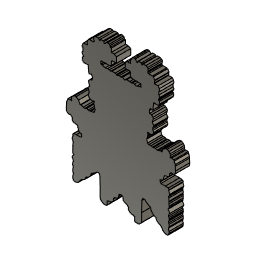
Keychain (Autodesk Fusion 360 design; units mm, degrees)
Autodesk Fusion 360 part; units mm, degrees
sketch "Sketch1" plane through (0, 0, 0) normal (0, 1, 0) x (1, 0, 0)
  line L0 (0.3, -15.5) -> (0.3, -15.9)
  line L1 (0.3, -15.9) -> (0.379, -15.9401)
  line L2 (0.379, -15.9401) -> (0.466, -15.9842)
  line L3 (0.466, -15.9842) -> (0.55, -15.9842)
  line L4 (0.55, -15.9842) -> (0.6648, -15.9842)
  line L5 (0.6648, -15.9842) -> (0.6648, -16.25)
  line L6 (0.6648, -16.25) -> (0.75, -16.25)
  line L7 (0.75, -16.25) -> (0.75, -16.3598)
  line L8 (0.75, -16.3598) -> (0.8165, -16.4115)
  line L9 (0.8165, -16.4115) -> (0.9263, -16.4405)
  line L10 (0.9263, -16.4405) -> (1.007, -16.426)
  line L11 (1.007, -16.426) -> (1.0561, -16.3628)
  line L12 (1.0561, -16.3628) -> (1.1168, -16.2847)
  line L13 (1.1168, -16.2847) -> (1.1655, -16.2759)
  line L14 (1.1655, -16.2759) -> (1.184, -16.3787)
  line L15 (1.184, -16.3787) -> (1.2314, -16.4034)
  line L16 (1.2314, -16.4034) -> (1.35, -16.4034)
  line L17 (1.35, -16.4034) -> (1.43, -16.4034)
  line L18 (1.43, -16.4034) -> (1.4623, -16.3414)
  line L19 (1.4623, -16.3414) -> (1.4623, -16.2775)
  line L20 (1.4623, -16.2775) -> (1.5139, -16.3414)
  line L21 (1.5139, -16.3414) -> (1.5602, -16.3987)
  line L22 (1.5602, -16.3987) -> (1.6237, -16.3987)
  line L23 (1.6237, -16.3987) -> (1.75, -16.3987)
  line L24 (1.75, -16.3987) -> (1.8659, -16.3356)
  line L25 (1.8659, -16.3356) -> (1.9094, -16.2678)
  line L26 (1.9094, -16.2678) -> (1.9094, -16.2)
  line L27 (1.9094, -16.2) -> (1.9094, -16.15)
  line L28 (1.9094, -16.15) -> (1.8726, -16.0823)
  line L29 (1.8726, -16.0823) -> (1.8726, -16.0289)
  line L30 (1.8726, -16.0289) -> (1.9342, -15.9953)
  line L31 (1.9342, -15.9953) -> (2.05, -15.9953)
  line L32 (2.05, -15.9953) -> (2.1322, -15.9953)
  line L33 (2.1322, -15.9953) -> (2.2162, -15.9953)
  line L34 (2.2162, -15.9953) -> (2.2759, -15.974)
  line L35 (2.2759, -15.974) -> (2.305, -15.9304)
  line L36 (2.305, -15.9304) -> (2.3387, -15.8797)
  line L37 (2.3387, -15.8797) -> (2.376, -15.8239)
  line L38 (2.376, -15.8239) -> (2.3574, -15.7715)
  line L39 (2.3574, -15.7715) -> (2.3574, -15.7205)
  line L40 (2.3574, -15.7205) -> (2.3574, -15.65)
  line L41 (2.3574, -15.65) -> (2.3381, -15.5959)
  line L42 (2.3381, -15.5959) -> (2.45, -15.5959)
  line L43 (2.45, -15.5959) -> (2.5213, -15.5959)
  line L44 (2.5213, -15.5959) -> (2.6101, -15.5959)
  line L45 (2.6101, -15.5959) -> (2.694, -15.4671)
  line L46 (2.694, -15.4671) -> (2.7215, -15.304)
  line L47 (2.7215, -15.304) -> (2.6654, -15.2946)
  line L48 (2.6654, -15.2946) -> (2.6654, -15.0651)
  line L49 (2.6654, -15.0651) -> (2.7369, -14.9554)
  line L50 (2.7369, -14.9554) -> (2.6654, -14.8407)
  line L51 (2.6654, -14.8407) -> (2.6201, -14.768)
  line L52 (2.6201, -14.768) -> (2.6428, -14.7332)
  line L53 (2.6428, -14.7332) -> (2.7012, -14.6968)
  line L54 (2.7012, -14.6968) -> (2.7012, -14.5195)
  line L55 (2.7012, -14.5195) -> (2.6315, -14.4076)
  line L56 (2.6315, -14.4076) -> (2.2904, -14.4076)
  line L57 (2.2904, -14.4076) -> (2.25, -13.95)
  line L58 (2.25, -13.95) -> (2.2, -13.9)
  line L59 (2.2, -13.9) -> (2.0693, -13.95)
  line L60 (2.0693, -13.95) -> (2.0337, -13.9)
  line L61 (2.0337, -13.9) -> (1.9883, -13.7813)
  line L62 (1.9883, -13.7813) -> (2.011, -13.6219)
  line L63 (2.011, -13.6219) -> (2.15, -13.6)
  line L64 (2.15, -13.6) -> (2.25, -13.5)
  line L65 (2.25, -13.5) -> (2.2661, -13.3873)
  line L66 (2.2661, -13.3873) -> (2.2387, -13.3159)
  line L67 (2.2387, -13.3159) -> (2.2, -13.2146)
  line L68 (2.2, -13.2146) -> (2.1861, -13.1782)
  line L69 (2.1861, -13.1782) -> (2.2524, -13.094)
  line L70 (2.2524, -13.094) -> (2.306, -13.026)
  line L71 (2.306, -13.026) -> (2.2792, -12.9559)
  line L72 (2.2792, -12.9559) -> (2.2524, -12.8986)
  line L73 (2.2524, -12.8986) -> (2.2192, -12.784)
  line L74 (2.2192, -12.784) -> (2.2524, -12.7162)
  line L75 (2.2524, -12.7162) -> (2.2926, -12.6016)
  line L76 (2.2926, -12.6016) -> (2.2524, -12.5047)
  line L77 (2.2524, -12.5047) -> (2.2358, -12.4648)
  line L78 (2.2358, -12.4648) -> (2.1355, -12.382)
  line L79 (2.1355, -12.382) -> (1.9902, -12.3659)
  line L80 (1.9902, -12.3659) -> (1.9111, -12.3987)
  line L81 (1.9111, -12.3987) -> (1.8582, -12.3928)
  line L82 (1.8582, -12.3928) -> (1.9111, -12.2707)
  line L83 (1.9111, -12.2707) -> (1.8582, -12.1463)
  line L84 (1.8582, -12.1463) -> (1.85, -12.05)
  line L85 (1.85, -12.05) -> (1.8058, -11.9463)
  line L86 (1.8058, -11.9463) -> (1.8582, -11.7379)
  line L87 (1.8582, -11.7379) -> (1.9596, -11.6947)
  line L88 (1.9596, -11.6947) -> (2.1, -11.6947)
  line L89 (2.1, -11.6947) -> (2.1978, -11.6531)
  line L90 (2.1978, -11.6531) -> (2.2806, -11.6739)
  line L91 (2.2806, -11.6739) -> (2.4147, -11.6947)
  line L92 (2.4147, -11.6947) -> (2.5352, -11.6434)
  line L93 (2.5352, -11.6434) -> (2.6372, -11.6691)
  line L94 (2.6372, -11.6691) -> (2.7893, -11.7347)
  line L95 (2.7893, -11.7347) -> (2.8635, -11.6947)
  line L96 (2.8635, -11.6947) -> (2.9118, -11.8081)
  line L97 (2.9118, -11.8081) -> (2.9653, -11.9337)
  line L98 (2.9653, -11.9337) -> (3.0346, -11.9801)
  line L99 (3.0346, -11.9801) -> (3.1448, -12.0537)
  line L100 (3.1448, -12.0537) -> (3.25, -12.0537)
  line L101 (3.25, -12.0537) -> (3.3107, -12.0169)
  line L102 (3.3107, -12.0169) -> (3.3771, -11.9766)
  line L103 (3.3771, -11.9766) -> (3.4512, -11.8816)
  line L104 (3.4512, -11.8816) -> (3.4738, -11.788)
  line L105 (3.4738, -11.788) -> (3.4625, -11.7153)
  line L106 (3.4625, -11.7153) -> (3.4512, -11.6427)
  line L107 (3.4512, -11.6427) -> (3.5563, -11.668)
  line L108 (3.5563, -11.668) -> (3.7193, -11.6427)
  line L109 (3.7193, -11.6427) -> (3.7352, -11.5769)
  line L110 (3.7352, -11.5769) -> (3.7805, -11.478)
  line L111 (3.7805, -11.478) -> (3.8142, -11.4044)
  line L112 (3.8142, -11.4044) -> (3.8142, -11.3)
  line L113 (3.8142, -11.3) -> (3.8305, -11.0228)
  line L114 (3.8305, -11.0228) -> (3.8142, -10.8387)
  line L115 (3.8142, -10.8387) -> (3.7, -10.75)
  line L116 (3.7, -10.75) -> (3.5622, -10.7419)
  line L117 (3.5622, -10.7419) -> (3.5425, -10.7672)
  line L118 (3.5425, -10.7672) -> (3.4401, -10.6876)
  line L119 (3.4401, -10.6876) -> (3.4076, -10.6159)
  line L120 (3.4076, -10.6159) -> (3.4137, -10.5115)
  line L121 (3.4137, -10.5115) -> (3.3672, -10.4448)
  line L122 (3.3672, -10.4448) -> (3.2816, -10.398)
  line L123 (3.2816, -10.398) -> (3.1846, -10.3923)
  line L124 (3.1846, -10.3923) -> (3.2816, -10.398)
  line L125 (3.05, -10.35) -> (3.1846, -10.3923)
  line L126 (3, -10.2) -> (3.05, -10.35)
  line L127 (3, -10.2) -> (2.9398, -10.0194)
  line L128 (2.9398, -10.0194) -> (2.7537, -9.9674)
  line L129 (2.7537, -9.9674) -> (2.7537, -9.8226)
  line L130 (2.7537, -9.8226) -> (2.8, -9.75)
  line L131 (2.8, -9.75) -> (2.95, -9.75)
  line L132 (2.95, -9.75) -> (3.1184, -9.75)
  line L133 (3.1184, -9.75) -> (3.3137, -9.7249)
  line L134 (3.3137, -9.7249) -> (3.387, -9.6621)
  line L135 (3.387, -9.6621) -> (3.3504, -9.5941)
  line L136 (3.3504, -9.5941) -> (3.387, -9.4947)
  line L137 (3.387, -9.4947) -> (3.4232, -9.3965)
  line L138 (3.4232, -9.3965) -> (3.387, -9.3294)
  line L139 (3.387, -9.3294) -> (3.3504, -9.2225)
  line L140 (3.3504, -9.2225) -> (3.3504, -9.1296)
  line L141 (3.3504, -9.1296) -> (3.3687, -9.0399)
  line L142 (3.3687, -9.0399) -> (3.3842, -8.964)
  line L143 (3.3842, -8.964) -> (3.3595, -8.8922)
  line L144 (3.3595, -8.8922) -> (3.3794, -8.7948)
  line L145 (3.3794, -8.7948) -> (3.3764, -8.8094)
  line L146 (3.3794, -8.6553) -> (3.3794, -8.5752)
  line L147 (3.3794, -8.5752) -> (3.3595, -8.4886)
  line L148 (3.3595, -8.4886) -> (3.3, -8.45)
  line L149 (3.3, -8.45) -> (3.3794, -8.3276)
  line L150 (3.3794, -8.3276) -> (3.4347, -8.2423)
  line L151 (3.4347, -8.2423) -> (3.3794, -8.1826)
  line L152 (3.3794, -8.1826) -> (3.3397, -8.0704)
  line L153 (3.3397, -8.0704) -> (3.3221, -8.0205)
  line L154 (3.3221, -8.0205) -> (3.3794, -7.9674)
  line L155 (3.3794, -7.9674) -> (3.3794, -7.8653)
  line L156 (3.3794, -7.8653) -> (3.4071, -7.8226)
  line L157 (3.4071, -7.8226) -> (3.3507, -7.7387)
  line L158 (3.3507, -7.7387) -> (3.3507, -7.6217)
  line L159 (3.3507, -7.6217) -> (3.3789, -7.556)
  line L160 (3.3789, -7.556) -> (3.3789, -7.4711)
  line L161 (3.3789, -7.4711) -> (3.3789, -7.4)
  line L162 (3.3789, -7.4) -> (3.3648, -7.3365)
  line L163 (3.3648, -7.3365) -> (3.3226, -7.2788)
  line L164 (3.3226, -7.2788) -> (3.3437, -7.2179)
  line L165 (3.3437, -7.2179) -> (3.3789, -7.1164)
  line L166 (3.3789, -7.1164) -> (3.3789, -7)
  line L167 (3.3789, -7) -> (3.3437, -6.9102)
  line L168 (3.3437, -6.9102) -> (3.3012, -6.8521)
  line L169 (3.3012, -6.8521) -> (3.2555, -6.8362)
  line L170 (3.2555, -6.8362) -> (3.1239, -6.8442)
  line L171 (3.1239, -6.8442) -> (3.0316, -6.8811)
  line L172 (3.0316, -6.8811) -> (2.95, -6.95)
  line L173 (2.95, -6.95) -> (2.9012, -7.0256)
  line L174 (2.9012, -7.0256) -> (2.863, -7.0846)
  line L175 (2.863, -7.0846) -> (2.8348, -7.1283)
  line L176 (2.8348, -7.1283) -> (2.75, -7.2)
  line L177 (2.75, -7.2) -> (2.65, -7.25)
  line L178 (2.65, -7.25) -> (2.55, -7.3)
  line L179 (2.55, -7.3) -> (2.4986, -7.3795)
  line L180 (2.4986, -7.3795) -> (2.4602, -7.4391)
  line L181 (2.4602, -7.4391) -> (2.4602, -7.5)
  line L182 (2.4602, -7.5) -> (2.3195, -7.5528)
  line L183 (2.3195, -7.5528) -> (2.1913, -7.6682)
  line L184 (2.1913, -7.6682) -> (2.1144, -7.7643)
  line L185 (2.1144, -7.7643) -> (2.0679, -7.9214)
  line L186 (2.0679, -7.9214) -> (1.9136, -8.0152)
  line L187 (1.9136, -8.0152) -> (1.787, -8.0923)
  line L188 (1.787, -8.0923) -> (1.6913, -8.1826)
  line L189 (1.6913, -8.1826) -> (1.593, -8.2104)
  line L190 (1.593, -8.2104) -> (1.5071, -8.1826)
  line L191 (1.5071, -8.1826) -> (1.4685, -8.0461)
  line L192 (1.4685, -8.0461) -> (1.45, -7.8)
  line L193 (1.45, -7.8) -> (1.4685, -8.0461)
  line L194 (1.45, -7.3) -> (1.45, -6.9)
  line L195 (1.45, -6.9) -> (1.45, -6.7)
  line L196 (1.45, -6.7) -> (1.3595, -6.593)
  line L197 (1.3595, -6.593) -> (1.25, -6.5)
  line L198 (1.25, -6.5) -> (1, -6.5)
  line L199 (1, -6.5) -> (0.9605, -6.5465)
  line L200 (0.9605, -6.5465) -> (0.9605, -6.6832)
  line L201 (0.9605, -6.6832) -> (0.9605, -6.8)
  line L202 (0.9605, -6.8) -> (0.85, -6.85)
  line L203 (0.85, -6.85) -> (0.75, -6.85)
  line L204 (0.75, -6.85) -> (0.6182, -6.9096)
  line L205 (0.6182, -6.9096) -> (0.5217, -6.9985)
  line L206 (0.5217, -6.9985) -> (0.5217, -7.15)
  line L207 (0.5217, -7.15) -> (0.45, -7.25)
  line L208 (0.45, -7.25) -> (0.3, -7.3)
  line L209 (0.3, -7.3) -> (0.15, -7.4)
  line L210 (0.15, -7.4) -> (0.15, -7.5)
  line L211 (0.15, -7.5) -> (0.1215, -7.6159)
  line L212 (0.1215, -7.6159) -> (0.0203, -7.6496)
  line L213 (0.0203, -7.6496) -> (-0.0016, -7.6569)
  line L214 (0.3, -15.5) -> (0.6, -15.5)
  line L215 (0.6, -15.5) -> (0.6623, -15.4533)
  line L216 (0.6623, -15.4533) -> (0.6623, -15.1993)
  line L217 (0.6623, -15.1993) -> (0.7687, -15.1197)
  line L218 (0.7687, -15.1197) -> (1.108, -15.1197)
  line L219 (1.108, -15.1197) -> (1.4, -15.1)
  line L220 (1.4, -15.1) -> (1.4, -14.9011)
  line L221 (1.4, -14.9011) -> (1.3, -14.9)
  line L222 (1.3, -14.9) -> (1.108, -14.8205)
  line L223 (1.108, -14.8205) -> (0.9383, -14.8603)
  line L224 (0.9383, -14.8603) -> (0.8, -14.8603)
  line L225 (0.8, -14.8603) -> (0.704, -14.8205)
  line L226 (0.704, -14.8205) -> (0.6222, -14.8603)
  line L227 (0.6222, -14.8603) -> (0.5, -14.8603)
  line L228 (0.5, -14.8603) -> (0.4, -14.8603)
  line L229 (0.4, -14.8603) -> (0.3075, -14.822)
  line L230 (0.3075, -14.822) -> (0.2833, -14.7721)
  line L231 (0.2833, -14.7721) -> (0.1019, -14.8603)
  line L232 (0.1019, -14.8603) -> (-0.0045, -14.8162)
  line L233 (-0.7839, -15.1197) -> (-1.1232, -15.1197)
  line L234 (-0.3152, -15.9) -> (-0.3942, -15.9401)
  line L235 (-2.5365, -15.5959) -> (-2.6253, -15.5959)
  line L236 (-2.3539, -15.8797) -> (-2.3912, -15.8239)
  line L237 (-2.2676, -12.8986) -> (-2.2344, -12.784)
  line L238 (-0.7652, -16.3598) -> (-0.8317, -16.4115)
  line L239 (-1.1992, -16.3787) -> (-1.2466, -16.4034)
  line L240 (-0.3227, -14.822) -> (-0.2985, -14.7721)
  line L241 (-1.0713, -16.3628) -> (-1.132, -16.2847)
  line L242 (-0.9757, -6.6832) -> (-0.9757, -6.8)
  line L243 (-0.8652, -6.85) -> (-0.7652, -6.85)
  line L244 (-0.4152, -14.8603) -> (-0.3227, -14.822)
  line L245 (-0.1171, -14.8603) -> (-0.0107, -14.8162)
  line L246 (-0.5369, -7.15) -> (-0.4652, -7.25)
  line L247 (-1.3747, -6.593) -> (-1.2652, -6.5)
  line L248 (-0.6775, -15.4533) -> (-0.6775, -15.1993)
  line L249 (-1.0222, -16.426) -> (-1.0713, -16.3628)
  line L250 (-1.4152, -14.9011) -> (-1.3152, -14.9)
  line L251 (-1.4775, -16.2775) -> (-1.5291, -16.3414)
  line L252 (-2.6806, -14.8407) -> (-2.6353, -14.768)
  line L253 (-0.68, -16.25) -> (-0.7652, -16.25)
  line L254 (-0.9757, -6.5465) -> (-0.9757, -6.6832)
  line L255 (-0.7652, -16.25) -> (-0.7652, -16.3598)
  line L256 (-1.4452, -16.4034) -> (-1.4775, -16.3414)
  line L257 (-1.1807, -16.2759) -> (-1.1992, -16.3787)
  line L258 (-0.1652, -7.5) -> (-0.1367, -7.6159)
  line L259 (-2.2314, -15.9953) -> (-2.2911, -15.974)
  line L260 (-1.1232, -14.8205) -> (-0.9535, -14.8603)
  line L261 (-1.3152, -14.9) -> (-1.1232, -14.8205)
  line L262 (-0.6374, -14.8603) -> (-0.5152, -14.8603)
  line L263 (-2.7092, -15.4671) -> (-2.7366, -15.304)
  line L264 (-0.5652, -15.9842) -> (-0.68, -15.9842)
  line L265 (-1.4152, -15.1) -> (-1.4152, -14.9011)
  line L266 (-0.6775, -15.1993) -> (-0.7839, -15.1197)
  line L267 (-0.1367, -7.6159) -> (-0.0355, -7.6496)
  line L268 (-0.3152, -15.5) -> (-0.6152, -15.5)
  line L269 (-2.9805, -11.9337) -> (-3.0498, -11.9801)
  line L270 (-1.0152, -6.5) -> (-0.9757, -6.5465)
  line L271 (-2.0844, -13.95) -> (-2.0489, -13.9)
  line L272 (-0.1652, -7.4) -> (-0.1652, -7.5)
  line L273 (-0.3942, -15.9401) -> (-0.4812, -15.9842)
  line L274 (-1.1232, -15.1197) -> (-1.4152, -15.1)
  line L275 (-2.3725, -15.7205) -> (-2.3725, -15.65)
  line L276 (-3.16, -12.0537) -> (-3.2652, -12.0537)
  line L277 (-0.7652, -6.85) -> (-0.6334, -6.9096)
  line L278 (-2.3056, -14.4076) -> (-2.2652, -13.95)
  line L279 (-1.8734, -12.1463) -> (-1.8652, -12.05)
  line L280 (-0.9415, -16.4405) -> (-1.0222, -16.426)
  line L281 (-2.3533, -15.5959) -> (-2.4652, -15.5959)
  line L282 (-1.2652, -6.5) -> (-1.0152, -6.5)
  line L283 (-2.927, -11.8081) -> (-2.9805, -11.9337)
  line L284 (-0.4812, -15.9842) -> (-0.5652, -15.9842)
  line L285 (-0.2985, -14.7721) -> (-0.1171, -14.8603)
  line L286 (-0.0355, -7.6496) -> (-0.0136, -7.6569)
  line L287 (-2.4652, -15.5959) -> (-2.5365, -15.5959)
  line L288 (-1.9246, -16.2) -> (-1.9246, -16.15)
  line L289 (-1.9246, -16.2678) -> (-1.9246, -16.2)
  line L290 (-2.2152, -13.2146) -> (-2.2013, -13.1782)
  line L291 (-3.8294, -11.3) -> (-3.8457, -11.0228)
  line L292 (-3.3659, -7.7387) -> (-3.3659, -7.6217)
  line L293 (-2.6524, -11.6691) -> (-2.8044, -11.7347)
  line L294 (-2.85, -7.1283) -> (-2.7652, -7.2)
  line L295 (-2.4753, -7.4391) -> (-2.4753, -7.5)
  line L296 (-2.2013, -13.1782) -> (-2.2676, -13.094)
  line L297 (-3.5714, -11.668) -> (-3.7345, -11.6427)
  line L298 (-3.7152, -10.75) -> (-3.5773, -10.7419)
  line L299 (-1.8734, -11.7379) -> (-1.9748, -11.6947)
  line L300 (-2.1296, -7.7643) -> (-2.0831, -7.9214)
  line L301 (-3.4289, -10.5115) -> (-3.3824, -10.4448)
  line L302 (-2.8152, -9.75) -> (-2.9652, -9.75)
  line L303 (-2.955, -10.0194) -> (-2.7689, -9.9674)
  line L304 (-2.213, -11.6531) -> (-2.2958, -11.6739)
  line L305 (-1.9263, -12.2707) -> (-1.8734, -12.1463)
  line L306 (-1.9288, -8.0152) -> (-1.8022, -8.0923)
  line L307 (-2.4299, -11.6947) -> (-2.5504, -11.6434)
  line L308 (-2.2539, -13.3159) -> (-2.2152, -13.2146)
  line L309 (-3.8294, -11.4044) -> (-3.8294, -11.3)
  line L310 (-3.3824, -10.4448) -> (-3.2968, -10.398)
  line L311 (-3.4227, -10.6159) -> (-3.4289, -10.5115)
  line L312 (-1.4652, -7.8) -> (-1.4836, -8.0461)
  line L313 (-3.7345, -11.6427) -> (-3.7504, -11.5769)
  line L314 (-2.5138, -7.3795) -> (-2.4753, -7.4391)
  line L315 (-2.2152, -13.9) -> (-2.0844, -13.95)
  line L316 (-3.3152, -8.45) -> (-3.3946, -8.3276)
  line L317 (-2.4753, -7.5) -> (-2.3347, -7.5528)
  line L318 (-2.0489, -13.9) -> (-2.0035, -13.7813)
  line L319 (-2.8044, -11.7347) -> (-2.8787, -11.6947)
  line L320 (-2.5652, -7.3) -> (-2.5138, -7.3795)
  line L321 (-2.1152, -11.6947) -> (-2.213, -11.6531)
  line L322 (-3.4889, -11.788) -> (-3.4776, -11.7153)
  line L323 (-3.0468, -6.8811) -> (-2.9652, -6.95)
  line L324 (-3.4663, -11.6427) -> (-3.5714, -11.668)
  line L325 (-3.7957, -11.478) -> (-3.8294, -11.4044)
  line L326 (-3.0152, -10.2) -> (-3.0652, -10.35)
  line L327 (-3.8294, -10.8387) -> (-3.7152, -10.75)
  line L328 (-3.8457, -11.0228) -> (-3.8294, -10.8387)
  line L329 (-2.6652, -7.25) -> (-2.5652, -7.3)
  line L330 (-2.7689, -9.8226) -> (-2.8152, -9.75)
  line L331 (-2.5504, -11.6434) -> (-2.6524, -11.6691)
  line L332 (-2.9164, -7.0256) -> (-2.8782, -7.0846)
  line L333 (-3.7504, -11.5769) -> (-3.7957, -11.478)
  line L334 (-1.5222, -8.1826) -> (-1.4836, -8.0461)
  line L335 (-2.9652, -6.95) -> (-2.9164, -7.0256)
  line L336 (-3.4553, -10.6876) -> (-3.4227, -10.6159)
  line L337 (-2.3347, -7.5528) -> (-2.2065, -7.6682)
  line L338 (-2.7652, -7.2) -> (-2.6652, -7.25)
  line L339 (-3.0152, -10.2) -> (-2.955, -10.0194)
  line L340 (-3.4776, -11.7153) -> (-3.4663, -11.6427)
  line L341 (-3.3747, -8.8922) -> (-3.3946, -8.7948)
  line L342 (-3.2968, -10.398) -> (-3.1998, -10.3923)
  line L343 (-2.7689, -9.9674) -> (-2.7689, -9.8226)
  line L344 (-2.3212, -13.026) -> (-2.2944, -12.9559)
  line L345 (-2.8782, -7.0846) -> (-2.85, -7.1283)
  line L346 (-0.5152, -14.8603) -> (-0.4152, -14.8603)
  line L347 (-0.6334, -6.9096) -> (-0.5369, -6.9985)
  line L348 (-0.4652, -7.25) -> (-0.3152, -7.3)
  line L349 (-1.9748, -11.6947) -> (-2.1152, -11.6947)
  line L350 (-2.2344, -12.784) -> (-2.2676, -12.7162)
  line L351 (-0.5369, -6.9985) -> (-0.5369, -7.15)
  line L352 (-1.132, -16.2847) -> (-1.1807, -16.2759)
  line L353 (-2.0262, -13.6219) -> (-2.1652, -13.6)
  line L354 (-2.0831, -7.9214) -> (-1.9288, -8.0152)
  line L355 (-0.7192, -14.8205) -> (-0.6374, -14.8603)
  line L356 (-3.3922, -11.9766) -> (-3.4663, -11.8816)
  line L357 (-1.2466, -16.4034) -> (-1.3652, -16.4034)
  line L358 (-0.3152, -7.3) -> (-0.1652, -7.4)
  line L359 (-0.68, -15.9842) -> (-0.68, -16.25)
  line L360 (-0.3152, -15.5) -> (-0.3152, -15.9)
  line L361 (-0.6152, -15.5) -> (-0.6775, -15.4533)
  line L362 (-1.9494, -15.9953) -> (-2.0652, -15.9953)
  line L363 (-0.8152, -14.8603) -> (-0.7192, -14.8205)
  line L364 (-2.1506, -12.382) -> (-2.0053, -12.3659)
  line L365 (-2.2676, -12.7162) -> (-2.3078, -12.6016)
  line L366 (-2.251, -12.4648) -> (-2.1506, -12.382)
  line L367 (-1.3652, -16.4034) -> (-1.4452, -16.4034)
  line L368 (-1.4652, -6.7) -> (-1.3747, -6.593)
  line L369 (-2.2065, -7.6682) -> (-2.1296, -7.7643)
  line L370 (-2.7164, -14.5195) -> (-2.6466, -14.4076)
  line L371 (-1.4836, -8.0461) -> (-1.4652, -7.8)
  line L372 (-2.6806, -15.2946) -> (-2.6806, -15.0651)
  line L373 (-2.3201, -15.9304) -> (-2.3539, -15.8797)
  line L374 (-2.6253, -15.5959) -> (-2.7092, -15.4671)
  line L375 (-1.821, -11.9463) -> (-1.8734, -11.7379)
  line L376 (-1.5754, -16.3987) -> (-1.6389, -16.3987)
  line L377 (-2.3725, -15.65) -> (-2.3533, -15.5959)
  line L378 (-2.6466, -14.4076) -> (-2.3056, -14.4076)
  line L379 (-1.8734, -12.3928) -> (-1.9263, -12.2707)
  line L380 (-3.4663, -11.8816) -> (-3.4889, -11.788)
  line L381 (-2.8787, -11.6947) -> (-2.927, -11.8081)
  line L382 (-3.3259, -12.0169) -> (-3.3922, -11.9766)
  line L383 (-3.0498, -11.9801) -> (-3.16, -12.0537)
  line L384 (-2.2911, -15.974) -> (-2.3201, -15.9304)
  line L385 (-2.3078, -12.6016) -> (-2.2676, -12.5047)
  line L386 (-1.7652, -16.3987) -> (-1.881, -16.3356)
  line L387 (-2.7521, -14.9554) -> (-2.6806, -14.8407)
  line L388 (-2.7164, -14.6968) -> (-2.7164, -14.5195)
  line L389 (-2.0035, -13.7813) -> (-2.0262, -13.6219)
  line L390 (-1.5291, -16.3414) -> (-1.5754, -16.3987)
  line L391 (-1.7065, -8.1826) -> (-1.6082, -8.2104)
  line L392 (-2.0652, -15.9953) -> (-2.1474, -15.9953)
  line L393 (-1.8652, -12.05) -> (-1.821, -11.9463)
  line L394 (-2.1474, -15.9953) -> (-2.2314, -15.9953)
  line L395 (-2.2652, -13.95) -> (-2.2152, -13.9)
  line L396 (-3.2652, -12.0537) -> (-3.3259, -12.0169)
  line L397 (-2.2676, -13.094) -> (-2.3212, -13.026)
  line L398 (-1.4775, -16.3414) -> (-1.4775, -16.2775)
  line L399 (-3.1391, -6.8442) -> (-3.0468, -6.8811)
  line L400 (-1.6082, -8.2104) -> (-1.5222, -8.1826)
  line L401 (-1.881, -16.3356) -> (-1.9246, -16.2678)
  line L402 (-2.658, -14.7332) -> (-2.7164, -14.6968)
  line L403 (-1.8877, -16.0823) -> (-1.8877, -16.0289)
  line L404 (-1.4652, -6.9) -> (-1.4652, -6.7)
  line L405 (-2.7366, -15.304) -> (-2.6806, -15.2946)
  line L406 (-2.1652, -13.6) -> (-2.2652, -13.5)
  line L407 (-1.8022, -8.0923) -> (-1.7065, -8.1826)
  line L408 (-1.9263, -12.3987) -> (-1.8734, -12.3928)
  line L409 (-1.9246, -16.15) -> (-1.8877, -16.0823)
  line L410 (-1.8877, -16.0289) -> (-1.9494, -15.9953)
  line L411 (-2.2812, -13.3873) -> (-2.2539, -13.3159)
  line L412 (-3.0652, -10.35) -> (-3.1998, -10.3923)
  line L413 (-2.2944, -12.9559) -> (-2.2676, -12.8986)
  line L414 (-2.2676, -12.5047) -> (-2.251, -12.4648)
  line L415 (-2.9652, -9.75) -> (-3.1335, -9.75)
  line L416 (-2.6806, -15.0651) -> (-2.7521, -14.9554)
  line L417 (-2.2652, -13.5) -> (-2.2812, -13.3873)
  line L418 (-1.6389, -16.3987) -> (-1.7652, -16.3987)
  line L419 (-2.3725, -15.7715) -> (-2.3725, -15.7205)
  line L420 (-2.0053, -12.3659) -> (-1.9263, -12.3987)
  line L421 (-1.4652, -7.3) -> (-1.4652, -6.9)
  line L422 (-2.3912, -15.8239) -> (-2.3725, -15.7715)
  line L423 (-2.6353, -14.768) -> (-2.658, -14.7332)
  line L424 (-2.2958, -11.6739) -> (-2.4299, -11.6947)
  line L425 (-0.9757, -6.8) -> (-0.8652, -6.85)
  line L426 (-0.8317, -16.4115) -> (-0.9415, -16.4405)
  line L427 (-0.9535, -14.8603) -> (-0.8152, -14.8603)
  line L428 (-3.1998, -10.3923) -> (-3.2968, -10.398)
  line L429 (-3.3941, -7.556) -> (-3.3941, -7.4711)
  line L430 (-3.4223, -7.8226) -> (-3.3659, -7.7387)
  line L431 (-3.38, -7.3365) -> (-3.3378, -7.2788)
  line L432 (-3.3378, -7.2788) -> (-3.3589, -7.2179)
  line L433 (-3.2707, -6.8362) -> (-3.1391, -6.8442)
  line L434 (-3.3946, -8.5752) -> (-3.3747, -8.4886)
  line L435 (-3.5773, -10.7419) -> (-3.5577, -10.7672)
  line L436 (-3.3656, -9.1296) -> (-3.3839, -9.0399)
  line L437 (-3.3589, -7.2179) -> (-3.3941, -7.1164)
  line L438 (-3.3946, -8.1826) -> (-3.3549, -8.0704)
  line L439 (-3.1335, -9.75) -> (-3.3289, -9.7249)
  line L440 (-3.3372, -8.0205) -> (-3.3946, -7.9674)
  line L441 (-3.4022, -9.3294) -> (-3.3656, -9.2225)
  line L442 (-3.3946, -8.7948) -> (-3.3916, -8.8094)
  line L443 (-3.3839, -9.0399) -> (-3.3994, -8.964)
  line L444 (-3.3289, -9.7249) -> (-3.4022, -9.6621)
  line L445 (-3.3946, -8.6553) -> (-3.3946, -8.5752)
  line L446 (-3.4022, -9.6621) -> (-3.3656, -9.5941)
  line L447 (-3.3941, -7.4) -> (-3.38, -7.3365)
  line L448 (-3.3946, -7.9674) -> (-3.3946, -7.8653)
  line L449 (-3.3941, -7.4711) -> (-3.3941, -7.4)
  line L450 (-3.3659, -7.6217) -> (-3.3941, -7.556)
  line L451 (-3.3163, -6.8521) -> (-3.2707, -6.8362)
  line L452 (-3.5577, -10.7672) -> (-3.4553, -10.6876)
  line L453 (-3.4384, -9.3965) -> (-3.4022, -9.3294)
  line L454 (-3.3994, -8.964) -> (-3.3747, -8.8922)
  line L455 (-3.4499, -8.2423) -> (-3.3946, -8.1826)
  line L456 (-3.3549, -8.0704) -> (-3.3372, -8.0205)
  line L457 (-3.3747, -8.4886) -> (-3.3152, -8.45)
  line L458 (-3.3946, -8.3276) -> (-3.4499, -8.2423)
  line L459 (-3.3941, -7.1164) -> (-3.3941, -7)
  line L460 (-3.3589, -6.9102) -> (-3.3163, -6.8521)
  line L461 (-3.3946, -7.8653) -> (-3.4223, -7.8226)
  line L462 (-3.4022, -9.4947) -> (-3.4384, -9.3965)
  line L463 (-3.3941, -7) -> (-3.3589, -6.9102)
  line L464 (-3.3656, -9.5941) -> (-3.4022, -9.4947)
  line L465 (-3.3656, -9.2225) -> (-3.3656, -9.1296)
  line L466 (-3.3916, -8.8094) -> (-3.3946, -8.6553)
  line L467 (-1.4836, -8.0461) -> (-1.4652, -7.3)
  line L468 (1.4685, -8.0461) -> (1.45, -7.3)
  line L469 (3.3764, -8.8094) -> (3.3794, -8.6553)
  line L470 (-0.0136, -7.6569) -> (-0.0016, -7.6569)
  line L471 (-0.0107, -14.8162) -> (-0.0045, -14.8162)
  point P0 (-0.0076, -16.5369)
  constraint vertical L0
  constraint parallel L1 L2
  constraint perpendicular L0 L3
  constraint perpendicular L0 L4
  constraint perpendicular L4 L5
  constraint perpendicular L5 L6
  constraint perpendicular L6 L7
  constraint perpendicular L8 L11
  constraint perpendicular L8 L12
  constraint parallel L10 L13
  constraint perpendicular L13 L14
  constraint horizontal L16
  constraint perpendicular L15 L18
  constraint perpendicular L17 L19
  constraint parallel L20 L21
  constraint perpendicular L19 L22
  constraint perpendicular L19 L23
  constraint perpendicular L23 L26
  constraint perpendicular L23 L27
  constraint perpendicular L24 L28
  constraint parallel L27 L29
  constraint perpendicular L28 L30
  constraint perpendicular L29 L31
  constraint perpendicular L29 L32
  constraint perpendicular L29 L33
  constraint parallel L35 L36
  constraint parallel L35 L37
  constraint perpendicular L34 L38
  constraint vertical L39
  constraint parallel L39 L40
  constraint parallel L38 L41
  constraint perpendicular L39 L42
  constraint perpendicular L39 L43
  constraint parallel L43 L44
  constraint perpendicular L46 L47
  constraint perpendicular L43 L48
  constraint parallel L45 L49
  constraint parallel L50 L51
  constraint parallel L49 L52
  constraint perpendicular L51 L53
  constraint vertical L54
  constraint perpendicular L53 L55
  constraint perpendicular L54 L56
  constraint perpendicular L59 L61
  constraint parallel L62 L65
  constraint perpendicular L59 L66
  constraint parallel L66 L67
  constraint parallel L67 L68
  constraint parallel L69 L70
  constraint parallel L67 L71
  constraint parallel L76 L77
  constraint perpendicular L76 L80
  constraint parallel L79 L81
  constraint parallel L83 L85
  constraint perpendicular L83 L87
  constraint horizontal L88
  constraint perpendicular L83 L89
  constraint perpendicular L86 L90
  constraint parallel L89 L92
  constraint parallel L90 L93
  constraint perpendicular L92 L96
  constraint perpendicular L92 L97
  constraint parallel L98 L99
  constraint horizontal L100
  constraint parallel L101 L102
  constraint parallel L105 L106
  constraint perpendicular L104 L107
  constraint perpendicular L106 L108
  constraint perpendicular L107 L109
  constraint parallel L110 L111
  constraint vertical L112
  constraint perpendicular L113 L116
  constraint perpendicular L115 L117
  constraint perpendicular L117 L118
  constraint perpendicular L116 L120
  constraint perpendicular L120 L123
  constraint parallel L123 L124
  constraint parallel L126 L127
  constraint vertical L129
  constraint horizontal L131
  constraint parallel L131 L132
  constraint parallel L136 L137
  constraint parallel L135 L138
  constraint vertical L140
  constraint parallel L141 L142
  constraint parallel L139 L143
  constraint parallel L141 L144
  constraint parallel L144 L145
  constraint vertical L146
  constraint perpendicular L148 L149
  constraint perpendicular L148 L150
  constraint parallel L152 L153
  constraint perpendicular L151 L154
  constraint vertical L155
  constraint parallel L150 L156
  constraint parallel L155 L158
  constraint parallel L158 L160
  constraint parallel L160 L161
  constraint parallel L164 L165
  constraint parallel L161 L166
  constraint parallel L163 L168
  constraint perpendicular L164 L169
  constraint parallel L173 L174
  constraint parallel L174 L175
  constraint parallel L177 L178
  constraint parallel L175 L179
  constraint parallel L179 L180
  constraint vertical L181
  constraint parallel L186 L187
  constraint perpendicular L189 L191
  constraint parallel L192 L193
  constraint vertical L194
  constraint perpendicular L195 L198
  constraint perpendicular L197 L199
  constraint parallel L195 L200
  constraint parallel L195 L201
  constraint horizontal L203
  constraint parallel L202 L204
  constraint vertical L206
  constraint parallel L206 L210
  constraint parallel L208 L212
  constraint perpendicular L0 L214
  constraint parallel L0 L216
  constraint parallel L215 L217
  constraint perpendicular L0 L218
  constraint perpendicular L218 L220
  constraint perpendicular L220 L224
  constraint parallel L222 L225
  constraint parallel L224 L227
  constraint parallel L227 L228
  constraint parallel L225 L229
  constraint perpendicular L226 L230
  constraint perpendicular L230 L231
  constraint parallel L229 L232
  constraint horizontal L470
  constraint horizontal L471
sketch "Sketch2" plane through (0, 0, 0) normal (0, 1, 0) x (-1, 0, 0)
extrude "Extrude1" add sketch "Sketch1" along normal blind 1
